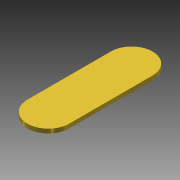
# Autodesk Inventor part: 13_1087_020
Saved by Autodesk Inventor 2014 (Build 180170000, 170)
## iProperties
Created: 2013-09-09
Part Number: 13_1087_020
Material: Allgemein
Document SubType Name: Modeling
Designer: vogel
Density: 1 g/cm^3
Appearance: Metall - 2400F (heiß)
Author: vogel
Autodesk Inventor part; units mm, degrees
ref_plane "YZ Plane" through (0, 0, 0) normal (1, 0, 0) x (0, 1, 0)
ref_plane "XZ Plane" through (0, 0, 0) normal (0, 1, 0) x (-1, 0, 0)
ref_plane "XY Plane" through (0, 0, 0) normal (0, 0, 1) x (1, 0, 0)
sketch "Skizze1" plane through (0, 0, 0) normal (0, 0, 1) x (1, 0, 0)
  line L0 (-3.5, 0) -> (3.5, 0) projected
  line L1 (0, -10.5) -> (0, 10.5) projected
  line L2 (0, 5) -> (0, -5) construction
  line L3 (2.5, 5) -> (2.5, -5)
  line L4 (-2.5, -5) -> (-2.5, 5)
  arc A0 (2.5, 5) -> (-2.5, 5) centre (0, 5) ccw
  arc A1 (-2.5, -5) -> (2.5, -5) centre (0, -5) ccw
  point P0 (0, 0)
  point P1 (0, 0)
  dimension "d0" = 15
  dimension "d1" = 5
  constraints: 8 end point, 4 point on circle, 4 tangent, 2 centre point, 2 point on line, 1 coincident, 1 midpoint, 1 parallel, 1 other
  measures "d1" distance between parallel lines of L3 L4
extrude "Extrusion1" add sketch "Skizze1" along normal blind 0.5
sketch "Skizze3" plane through (0, 0, 0) normal (0, 0, -1) x (-1, 0, 0)
  line L0 (-2.5, 5) -> (-2.5, -5) projected
  line L1 (0, -1.5) -> (0, 1.5) construction
  line L2 (1.5, -1.5) -> (1.5, 1.5)
  line L3 (-1.5, 1.5) -> (-1.5, -1.5)
  arc A0 (-1.5, -1.5) -> (1.5, -1.5) centre (0, -1.5) ccw
  arc A1 (1.5, 1.5) -> (-1.5, 1.5) centre (0, 1.5) ccw
  point P0 (0, 0)
  point P1 (0, 0)
  dimension "d8" = 3
  dimension "d9" = 6
  constraints: 8 end point, 4 point on circle, 4 tangent, 2 centre point, 2 parallel, 1 coincident, 1 midpoint
  measures "d8" distance between parallel lines of L2 L3
extrude "Extrusion3" cut sketch "Skizze3" against normal blind 0.2
